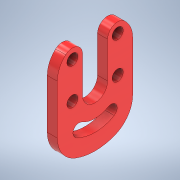
# Autodesk Inventor part: hw7
Saved by Autodesk Inventor 2021 (Build 250183000, 183)
## iProperties
Created: 2022-04-30
Part Number: hw7
Material: Generic
Document SubType Name: Modeling
Designer: authe
Density: 1 g/cm^3
Appearance: Light Red
Author: authe
Autodesk Inventor part; units mm, degrees
ref_plane "YZ Plane" through (0, 0, 0) normal (1, 0, 0) x (0, 1, 0)
ref_plane "XZ Plane" through (0, 0, 0) normal (0, 1, 0) x (-1, 0, 0)
ref_plane "XY Plane" through (0, 0, 0) normal (0, 0, 1) x (1, 0, 0)
sketch "Sketch1" plane through (0, 0, 0) normal (1, 0, 0) x (0, 1, 0)
  arc A0 (-50.2663, 19.7308) -> (-50.2663, -19.7308) centre (0, 0) ccw
  line L0 (24.8197, 37.5) -> (-24.2023, 37.5)
  line L1 (-24.2023, -37.5) -> (24.8197, -37.5)
  arc A1 (0, 12.5) -> (0, -12.5) centre (0, 0) ccw
  circle A2 centre (0, -22.5) radius 5.5
  circle A3 centre (0, 22.5) radius 5.5
  arc A4 (-24.2023, 37.5) -> (-50.2663, 19.7308) centre (-24.2023, 9.5) ccw
  line L2 (-14, 0) -> (-38, 0)
  arc A5 (-50.2663, -19.7308) -> (-24.2023, -37.5) centre (-24.2023, -9.5) ccw
  arc A6 (-22.5167, 13) -> (-32.909, 19) centre (-27.7128, 16) ccw
  arc A7 (-32.909, -19) -> (-22.5167, -13) centre (-27.7128, -16) ccw
  arc A8 (-32.909, 19) -> (-32.909, -19) centre (0, 0) ccw
  arc A9 (36, 12.5) -> (43.4536, 29.1667) centre (36, 22.5) ccw
  arc A10 (43.4536, -29.1667) -> (36, -12.5) centre (36, -22.5) ccw
  line L3 (0, 12.5) -> (0, -12.5)
  arc A11 (3.9746, 26.3016) -> (3.6179, 25.7471) centre (24.8197, 12.5) ccw
  arc A12 (-0.1803, 12.4987) -> (0, 9.5026) centre (24.8197, 12.5) ccw
  arc A13 (24.8197, -37.5) -> (43.4536, -29.1667) centre (24.8197, -12.5) ccw
  arc A14 (0, -9.5026) -> (-0.1803, -12.4987) centre (24.8197, -12.5) ccw
  arc A15 (43.4536, 29.1667) -> (24.8197, 37.5) centre (24.8197, 12.5) ccw
  line L4 (0, 12.5) -> (36, 12.5)
  line L5 (0, -12.5) -> (36, -12.5)
  circle A16 centre (36, 22.5) radius 5.5
  circle A17 centre (36, -22.5) radius 5.5
  arc A18 (-22.5167, 13) -> (-22.5167, -13) centre (0, 0) ccw
  dimension "d21" = 11
  dimension "d12" = 20
  dimension "d19" = 25
  dimension "d22" = 11
  dimension "d23" = 11
  dimension "d24" = 36
  dimension "d25" = 32
  dimension "d26" = 6
  constraints: 33 point on circle, 18 centre point, 12 end point, 4 coincident, 4 point on line, 4 tangent, 3 horizontal, 3 symmetric about line, 1 parallel, 1 vertical, 4 other
  measures "d12" diameter of A9
  measures "d19" diameter of A1
  measures "d22" diameter of A2
  measures "d23" diameter of A17
  measures "d24" distance of L3.start L4.end
  measures "d25" distance of A7.centre A6.centre
  measures "d26" radius of A6
extrude "Extrusion1" add sketch "Sketch1" along normal mid plane 10 contours A4 L0 A15 A9 L4 A1 L5 A10 A13 L1 A5 A0
body "Solid1"
